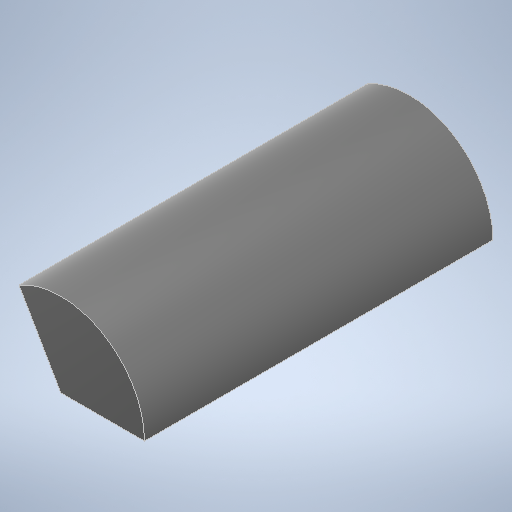
# Autodesk Inventor part: Epoxy
Saved by Autodesk Inventor 2026.2 (Build 302298010, 298A)
## iProperties
Created: 2026-04-26
Part Number: Epoxy
Material: Acetal Resin, Black
Document SubType Name: Modeling
Designer: piete
Density: 1.425 g/cm^3
Appearance: Smooth - Black
Author: piete
Autodesk Inventor part; units mm, degrees
ref_plane "YZ Plane" through (0, 0, 0) normal (1, 0, 0) x (0, 1, 0)
ref_plane "XZ Plane" through (0, 0, 0) normal (0, 1, 0) x (-1, 0, 0)
ref_plane "XY Plane" through (0, 0, 0) normal (0, 0, 1) x (1, 0, 0)
sketch "Sketch1" plane through (0, 0, 0) normal (0, 0, 1) x (1, 0, 0)
  line L0 (0, 0) -> (1.2, 0)
  line L1 (0, 0) -> (-0.6, 1.0392)
  line L2 (0, 0) -> (1.2, 0) construction
  circle A0 centre (0, 0) radius 1.2
  dimension "d0" = 1.2
  dimension "d1" = 1.2
  dimension "d2" = 120
  dimension "d3" = 2.4
  constraints: 6 end point, 2 horizontal, 1 centre point, 1 coincident, 1 equal length
  measures "d0" distance of L0.start L0.end
  measures "d1" distance of L0.start L1.end
  measures "d2" angle of L2 L1
  measures "d3" diameter of A0
extrude "Extrusion1" add sketch "Sketch1" along normal blind 5 contours L1 A0 L0 picked at (-0.138, 0.7825)
body "Solid1"
